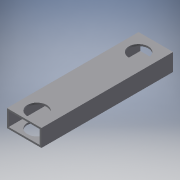
# Autodesk Inventor part: New intake
Saved by Autodesk Inventor 2018 (Build 220112000, 112)
## iProperties
Created: 2018-02-18
Part Number: New intake
Material: Generic
Document SubType Name: Modeling
Designer: Luke
Density: 1 g/cm^3
Appearance: Default
Author: Luke
Autodesk Inventor part; units mm, degrees
ref_plane "YZ Plane" through (0, 0, 0) normal (1, 0, 0) x (0, 1, 0)
ref_plane "XZ Plane" through (0, 0, 0) normal (0, 1, 0) x (-1, 0, 0)
ref_plane "XY Plane" through (0, 0, 0) normal (0, 0, 1) x (1, 0, 0)
sketch "Sketch1" plane through (0, 0, 0) normal (0, 0, 1) x (1, 0, 0)
  line L0 (0, 0) -> (50.8, 0)
  line L1 (50.8, 0) -> (50.8, -25.4)
  line L2 (50.8, -25.4) -> (0, -25.4)
  line L3 (0, -25.4) -> (0, 0)
  line L4 (48.26, -2.54) -> (2.54, -2.54)
  line L5 (2.54, -2.54) -> (2.54, -22.86)
  line L6 (2.54, -22.86) -> (48.26, -22.86)
  line L7 (48.26, -22.86) -> (48.26, -2.54)
  dimension "d0" = 50.8
  dimension "d1" = 25.4
  dimension "d2" = 2.54
  constraints: 16 end point, 4 parallel, 2 perpendicular, 1 horizontal, 3 other
  measures "d0" distance of L1.end L2.end
  measures "d1" distance of L0.end L1.end
  measures "d2" distance between parallel lines of L0 L4
extrude "Extrusion1" add sketch "Sketch1" along normal blind 168.275
sketch "Sketch2" plane through (0, 0, 0) normal (0, 1, 0) x (1, 0, 0)
  circle A0 centre (25.4, -25.4) radius 14.2875
  circle A1 centre (25.4, -149.225) radius 14.2875
  line L0 (50.8, 0) -> (50.8, -168.275) projected
  line L1 (50.8, -168.275) -> (0, -168.275) projected
  line L2 (0, 0) -> (50.8, 0) projected
  line L3 (0, 0) -> (0, -168.275) projected
  dimension "d5" = 25.4
  dimension "d6" = 19.05
  dimension "d7" = 25.4
  dimension "d8" = 25.4
  dimension "d9" = 28.575
  dimension "d10" = 28.575
  constraints: 2 centre point
  measures "d5" distance from line of L0 A1.centre
  measures "d6" distance from line of L1 A1.centre
  measures "d7" distance from line of L2 A0.centre
  measures "d8" distance from line of L3 A0.centre
  measures "d9" diameter of A0
  measures "d10" diameter of A1
extrude "Extrusion2" cut sketch "Sketch2" against normal blind 168.275 contours A0 | A1
body "Solid1"
